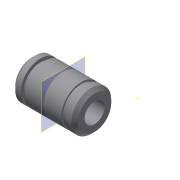
# Autodesk Inventor part: 00_IGUS_Drylin_RJ4JP-01-06
Saved by Autodesk Inventor 2019.4 (Build 234330000, 330)
## iProperties
Created: 2020-01-07
Part Number: 00_IGUS_Drylin_RJ4JP-01-06
Material: Generic
Document SubType Name: Modeling
Designer: diederichbenedict
Density: 1 g/cm^3
Appearance: Default
Author: diederichbenedict
Autodesk Inventor part; units mm, degrees
ref_plane "YZ Plane" through (0, 0, 0) normal (1, 0, 0) x (0, 1, 0)
ref_plane "XZ Plane" through (0, 0, 0) normal (0, 1, 0) x (-1, 0, 0)
ref_plane "XY Plane" through (0, 0, 0) normal (0, 0, 1) x (1, 0, 0)
sketch "Sketch1" plane through (0, 0, 0) normal (0, 1, 0) x (-1, 0, 0)
  line L0 (0, 254.7362) -> (18.9, 254.7362)
  line L1 (0, 254.7362) -> (18.9, 254.7362) construction
  line L2 (18.9, 254.7362) -> (18.9, 248.7362)
  line L3 (18.9, 248.7362) -> (16.3, 248.7362)
  line L4 (16.3, 248.7362) -> (16.3, 249.7362)
  line L5 (16.3, 249.7362) -> (15.1, 249.7362)
  line L6 (15.1, 249.7362) -> (15.1, 248.7362)
  line L7 (0, 254.7362) -> (0, 248.7362)
  line L8 (0, 248.7362) -> (2.8, 248.7362)
  line L9 (2.8, 248.7362) -> (2.8, 249.2362)
  line L10 (2.8, 249.2362) -> (4, 249.2362)
  line L11 (4, 249.2362) -> (4, 248.7362)
  line L12 (4, 248.7362) -> (15.1, 248.7362)
  line L13 (18.9, 251.7362) -> (0, 251.7362)
  point P0 (0, 0)
  dimension "d0" = 18.9
  dimension "d1" = 0
  dimension "d2" = 6
  dimension "d3" = 2.6
  dimension "d4" = 1
  dimension "d5" = 1.2
  dimension "d6" = 2.8
  dimension "d7" = 1.2
  dimension "d8" = 3
  constraints: 28 end point, 11 perpendicular, 2 horizontal, 2 midpoint, 2 point on line, 1 collinear, 1 vertical
  measures "d0" distance of L0.start L0.end
  measures "d1" distance between parallel lines of L0 L1
  measures "d2" distance of L0.end L2.end
  measures "d3" distance of L2.end L3.end
  measures "d4" distance of L3.end L4.end
  measures "d5" distance of L4.end L5.end
  measures "d6" distance of L7.end L8.end
  measures "d7" distance of L9.end L10.end
  measures "d8" distance between parallel lines of L13 L0
revolve "Revolution1" add sketch "Sketch1" angle 360 about axis through (0, 0, 254.7362) along (-1, 0, 0) contours L13 L2 L3 L4 L5 L6 L12 L11 L10 L9 L8 L7
chamfer "Chamfer1" distance 1 angle 45 2 edges at (0, 0, 260.7362) (-18.9, 0, 260.7362)
ref_plane "Work Plane1" through (-9.45, 0, 254.7362) normal (-1, 0, 0) x (0, 0, 1)
ref_plane "Work Plane2" through (-27.2784, 6.1407, 239.852) normal (0, -0.3924921, 0.9197554) x (1, 0, 0)
ref_plane "Work Plane3" through (-73.6784, -13.5496, 235.0374) normal (0, 0.9197554, 0.3924921) x (1, 0, 0)
body "Solid1"
